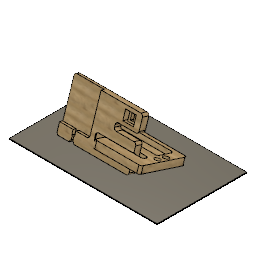
Phone Stand Valet Thingy (Autodesk Fusion 360 design; units mm, degrees)
Autodesk Fusion 360 part; units mm, degrees
note: some values were not read from the file. Set by a fixed rule: which sketch regions a step uses.
sketch "Face Plate Sketch" plane through (0, 0, 0) normal (0, 0, 1) x (1, 0, 0)
  line L0 (6.35, 0) -> (196.85, 0)
  line L1 (196.85, 136.525) -> (6.35, 136.525)
  line L2 (0, 130.175) -> (0, 6.35)
  line L3 (0, 28.575) -> (77.7875, 28.575)
  line L4 (84.1375, 34.925) -> (84.1375, 136.525)
  line L5 (196.85, 92.075) -> (146.05, 92.075)
  line L6 (139.7, 92.075) -> (139.7, 136.525)
  line L7 (139.7, 85.725) -> (139.7, 79.375)
  line L8 (146.05, 73.025) -> (196.85, 73.025)
  line L9 (203.2, 50.165) -> (103.1875, 50.165)
  line L10 (96.8375, 43.815) -> (96.8375, 34.925)
  line L11 (103.1875, 28.575) -> (203.2, 28.575)
  line L12 (203.2, 6.35) -> (203.2, 66.675)
  line L13 (203.2, 98.425) -> (203.2, 130.175)
  arc A0 (146.05, 92.075) -> (139.7, 85.725) centre (146.05, 85.725) ccw
  arc A1 (196.85, 92.075) -> (203.2, 98.425) centre (196.85, 98.425) ccw
  arc A2 (203.2, 130.175) -> (196.85, 136.525) centre (196.85, 130.175) ccw
  arc A3 (139.7, 79.375) -> (146.05, 73.025) centre (146.05, 79.375) ccw
  arc A4 (203.2, 66.675) -> (196.85, 73.025) centre (196.85, 66.675) ccw
  arc A5 (103.1875, 50.165) -> (96.8375, 43.815) centre (103.1875, 43.815) ccw
  arc A6 (96.8375, 34.925) -> (103.1875, 28.575) centre (103.1875, 34.925) ccw
  arc A7 (196.85, 0) -> (203.2, 6.35) centre (196.85, 6.35) ccw
  arc A8 (0, 6.35) -> (6.35, 0) centre (6.35, 6.35) ccw
  arc A9 (6.35, 136.525) -> (0, 130.175) centre (6.35, 130.175) ccw
  arc A10 (77.7875, 28.575) -> (84.1375, 34.925) centre (77.7875, 34.925) ccw
  line L14 (139.7, 114.3) -> (171.45, 114.3) construction
  line L15 (171.45, 92.075) -> (171.45, 127) construction
  line L16 (171.45, 114.3) -> (203.2, 114.3) construction
  line L17 (175.4188, 122.2375) -> (167.4813, 122.2375)
  line L18 (167.4813, 122.2375) -> (167.4813, 106.3625)
  line L19 (167.4813, 106.3625) -> (175.4188, 106.3625)
  line L20 (175.4188, 106.3625) -> (175.4188, 122.2375)
  line L21 (175.4188, 122.2375) -> (167.4813, 106.3625) construction
  line L22 (167.4813, 122.2375) -> (175.4188, 106.3625) construction
  line L23 (181.3719, 103.1875) -> (161.5281, 103.1875)
  line L24 (161.5281, 103.1875) -> (161.5281, 125.4125)
  line L25 (161.5281, 125.4125) -> (181.3719, 125.4125)
  line L26 (181.3719, 125.4125) -> (181.3719, 103.1875)
  line L27 (181.3719, 103.1875) -> (161.5281, 125.4125) construction
  line L28 (161.5281, 103.1875) -> (181.3719, 125.4125) construction
  line L29 (186.5313, 101.2031) -> (156.3688, 101.2031)
  line L30 (156.3688, 101.2031) -> (156.3688, 127.3969)
  line L31 (156.3688, 127.3969) -> (186.5313, 127.3969)
  line L32 (186.5313, 127.3969) -> (186.5313, 101.2031)
  line L33 (186.5313, 101.2031) -> (156.3688, 127.3969) construction
  line L34 (156.3688, 101.2031) -> (186.5313, 127.3969) construction
  line L35 (161.5281, 125.4125) -> (161.5281, 127.3969)
  line L36 (181.3719, 125.4125) -> (181.3719, 127.3969)
  line L37 (181.3719, 103.1875) -> (181.3719, 101.2031)
  line L38 (161.5281, 103.1875) -> (161.5281, 101.2031)
  line L39 (42.0687, 31.8116) -> (42.0687, 28.575) construction
  line L40 (38.1, 28.575) -> (46.0375, 28.575)
  line L41 (46.0375, 28.575) -> (46.0375, 16.6687)
  line L42 (46.0375, 16.6687) -> (38.1, 16.6687)
  line L43 (38.1, 16.6687) -> (38.1, 28.575)
  line L44 (44.2531, 16.6687) -> (39.8843, 16.6687)
  line L45 (39.8843, 16.6687) -> (39.8843, 5.5562)
  line L46 (39.8843, 5.5562) -> (44.2531, 5.5562)
  line L47 (44.2531, 5.5562) -> (44.2531, 16.6687)
  line L48 (40.4812, 5.5562) -> (43.6562, 5.5562)
  line L49 (43.6562, 5.5562) -> (43.6563, 0)
  line L50 (43.6563, 0) -> (40.4813, 0)
  line L51 (40.4813, 0) -> (40.4812, 5.5562)
  line L52 (40.4813, 0) -> (43.6563, 0)
  circle A11 centre (42.0688, 0) radius 6.35
  point P0 (203.2, 0)
  point P1 (84.1375, 28.575)
  point P2 (139.7, 73.025)
  point P3 (96.8375, 50.165)
  point P4 (96.8375, 28.575)
  point P5 (171.45, 114.3)
  point P6 (171.45, 114.3)
  point P7 (171.45, 114.3)
  point P8 (171.45, 114.3)
  point P9 (42.0687, 28.575)
  point P10 (42.0687, 16.6687)
  point P11 (42.0687, 16.6687)
  point P12 (42.0687, 5.5562)
  point P13 (42.0687, 5.5562)
  point P14 (42.0688, 0)
  dimension "d3" = 84.1375
  dimension "d5" = 44.45
  dimension "d6" = 19.05
  dimension "d8" = 12.7
  dimension "d9" = 21.59
  dimension "d12" = 28.575
  dimension "d13" = 25.4
  dimension "d28" = 6.35
  dimension "d29" = 6.35
  dimension "d30" = 6.35
  dimension "d31" = 6.35
  dimension "d32" = 6.35
  dimension "d33" = 6.35
  dimension "d76" = 106.3625
  dimension "d77" = 203.2
  dimension "d163" = 6.35
  dimension "d185" = 63.5
  dimension "d193" = 7.9375
  dimension "d194" = 15.875
  dimension "d195" = 19.8438
  dimension "d196" = 22.225
  dimension "d197" = 26.1938
  dimension "d198" = 30.1625
  dimension "d202" = 7.9375
  dimension "d203" = 11.9062
  dimension "d204" = 11.1125
  dimension "d205" = 4.3688
  dimension "d206" = 3.175
  dimension "d220" = 12.7
  dimension "d224" = 136.525
  measures "d3" distance of L3.start P1
  measures "d5" distance of L6.start L6.end
  measures "d6" distance of L6.start P2
  measures "d8" distance of L4 L10
  measures "d9" distance of P3 P4
  measures "d12" distance of L0 L11
  measures "d28" radius of A0
  measures "d29" radius of A1
  measures "d30" radius of A3
  measures "d31" radius of A5
  measures "d32" radius of A7
  measures "d33" radius of A10
  measures "d76" distance of L10 L12
  measures "d77" distance of L2 L12
  measures "d163" radius of A9
  measures "d185" distance of L6 L13
  measures "d193" distance of L17.start L17.end
  measures "d194" distance of L17.end L18.end
  measures "d195" distance of L24.end L25.end
  measures "d196" distance of L23.end L24.end
  measures "d197" distance of L29.end L30.end
  measures "d198" distance of L30.end L31.end
  measures "d202" distance of L40.start L40.end
  measures "d203" distance of L40.start L42.end
  measures "d204" distance of L44.start L46.end
  measures "d205" distance of L44.start L44.end
  measures "d206" distance of L48.start L48.end
  measures "d220" diameter of A11
  measures "d224" distance of L0 L1
extrude "Extrude1" add sketch "Face Plate Sketch" along normal blind 19.05 contours L0 L2 L3 A8 L42 L43 L45 A11 | L0 L1 L3 L4 L5 L7 L8 L9 L10 L11 L12 L13 A0 A1 A2 A3 A4 A5 A6 A7 A10 L41 L42 L47 A11 makes body 1 at (108.7286, 91.0847, 0) makes body 2 at (12.7, 17.1979, 0) in component "Face Plate"
extrude "Extrude6" add sketch "Face Plate Sketch" along normal blind 9.525 contours L42 L44 L45 L47 A11 | L3 L40 L41 L42 L43 L44 bodies 1 2 in component "Face Plate"
extrude "Extrude2" add sketch "Face Plate Sketch" along normal blind 15.875 contours L9 L10 L11 L12 A5 A6 bodies 1 in component "Face Plate"
extrude "Extrude4" add sketch "Face Plate Sketch" along normal blind 9.525 contours L1 L2 L3 L4 A9 A10 L40 bodies 1 in component "Face Plate"
extrude "Extrude5" add sketch "Face Plate Sketch" along normal blind 10.16 contours L23 L29 L37 L38 | L23 L24 L25 L26 | L25 L31 L35 L36 bodies 1 in component "Face Plate"
sketch "iPhone" plane through (0, 0, 0) normal (0, 0, 1) x (1, 0, 0)
  line L0 (0, 0) -> (77.724, 0)
  line L1 (77.724, 0) -> (77.724, 157.988)
  line L2 (77.724, 157.988) -> (0, 157.988)
  line L3 (0, 157.988) -> (0, 0)
  dimension "d49" = 157.988
  dimension "d50" = 77.724
  measures "d49" distance of L0.start L2.end
  measures "d50" distance of L1.end L2.end
extrude "Extrude1'" add sketch "iPhone" along normal blind 7.112 separate body makes body 3 in component "iPhone"
sketch "Base Plate Sketch" plane through (0, 0, 0) normal (0, 1, 0) x (1, 0, 0)
  line L0 (0, 0) -> (119.0625, 0)
  line L1 (125.4125, 6.35) -> (125.4125, 130.175)
  line L2 (119.0625, 136.525) -> (-71.4375, 136.525)
  line L3 (-6.35, 31.75) -> (93.6625, 31.75)
  line L4 (100.0125, 38.1) -> (100.0125, 42.8625)
  line L5 (93.6625, 49.2125) -> (-71.4375, 49.2125)
  arc A0 (93.6625, 31.75) -> (100.0125, 38.1) centre (93.6625, 38.1) ccw
  arc A1 (100.0125, 42.8625) -> (93.6625, 49.2125) centre (93.6625, 42.8625) ccw
  line L6 (-77.7875, 130.175) -> (-77.7875, 55.5625)
  line L7 (-6.35, 31.75) -> (-6.35, 6.35)
  circle A2 centre (112.7125, 87.3125) radius 7.9375
  arc A3 (-6.35, 6.35) -> (0, 0) centre (0, 6.35) ccw
  arc A4 (119.0625, 0) -> (125.4125, 6.35) centre (119.0625, 6.35) ccw
  arc A5 (125.4125, 130.175) -> (119.0625, 136.525) centre (119.0625, 130.175) ccw
  arc A6 (-71.4375, 136.525) -> (-77.7875, 130.175) centre (-71.4375, 130.175) ccw
  arc A7 (-77.7875, 55.5625) -> (-71.4375, 49.2125) centre (-71.4375, 55.5625) ccw
  line L8 (-58.7375, 123.825) -> (93.6625, 123.825)
  line L9 (100.0125, 117.475) -> (100.0125, 80.9625)
  line L10 (93.6625, 74.6125) -> (-58.7375, 74.6125)
  line L11 (-65.0875, 80.9625) -> (-65.0875, 117.475)
  arc A8 (-58.7375, 123.825) -> (-65.0875, 117.475) centre (-58.7375, 117.475) ccw
  arc A9 (-65.0875, 80.9625) -> (-58.7375, 74.6125) centre (-58.7375, 80.9625) ccw
  arc A10 (93.6625, 74.6125) -> (100.0125, 80.9625) centre (93.6625, 80.9625) ccw
  arc A11 (100.0125, 117.475) -> (93.6625, 123.825) centre (93.6625, 117.475) ccw
  line L12 (112.7125, 61.9125) -> (112.7125, 87.3125) construction
  line L13 (9.525, 65.8813) -> (25.4, 65.8813)
  line L14 (25.4, 65.8813) -> (25.4, 57.9438)
  line L15 (25.4, 57.9438) -> (9.525, 57.9438)
  line L16 (9.525, 57.9438) -> (9.525, 65.8813)
  line L17 (17.4625, 65.8813) -> (17.4625, 74.6125) construction
  line L18 (17.4625, 57.9438) -> (17.4625, 49.2125) construction
  arc A12 (112.4188, 69.8446) -> (113.0062, 53.9804) centre (112.7125, 61.9125) ccw
  arc A13 (113.0062, 53.9804) -> (112.4188, 69.8446) centre (112.7125, 61.9125) ccw
  line L19 (85.4474, 49.2125) -> (85.4474, 74.6125) construction
  line L20 (85.4474, 61.9125) -> (125.4125, 61.9125) construction
  point P0 (125.4125, 0)
  point P1 (125.4125, 136.525)
  point P2 (-77.7875, 136.525)
  point P3 (100.0125, 31.75)
  point P4 (17.4625, 74.6125)
  point P5 (17.4625, 65.8813)
  dimension "d80" = 17.4625
  dimension "d82" = 31.75
  dimension "d83" = 6.35
  dimension "d84" = 6.35
  dimension "d114" = 136.525
  dimension "d115" = 203.2
  dimension "d116" = 25.4
  dimension "d118" = 106.3625
  dimension "d143" = 15.875
  dimension "d144" = 12.7
  dimension "d146" = 6.35
  dimension "d147" = 6.35
  dimension "d148" = 6.35
  dimension "d149" = 6.35
  dimension "d150" = 6.35
  dimension "d151" = 12.7
  dimension "d152" = 25.4
  dimension "d153" = 12.7
  dimension "d154" = 25.4
  dimension "d156" = 6.35
  dimension "d157" = 6.35
  dimension "d158" = 6.35
  dimension "d159" = 6.35
  dimension "d201" = 15.875
  dimension "d221" = 15.875
  dimension "d222" = 7.9375
  dimension "d223" = 25.4
  measures "d80" distance of L3 L5
  measures "d82" distance of L0 L3
  measures "d83" radius of A0
  measures "d84" radius of A1
  measures "d114" distance of P0 P1
  measures "d115" distance of P1 P2
  measures "d116" distance of L1 L4
  measures "d118" distance of L4.end L7
  measures "d143" diameter of A2
  measures "d144" distance of L1 A2.centre
  measures "d146" radius of A3
  measures "d147" radius of A4
  measures "d148" radius of A5
  measures "d149" radius of A6
  measures "d150" radius of A7
  measures "d151" distance of L6 L11
  measures "d152" distance of L1 L9
  measures "d153" distance of L2 L8
  measures "d154" distance of L5 L10
  measures "d156" radius of A8
  measures "d157" radius of A9
  measures "d158" radius of A10
  measures "d159" radius of A11
  measures "d201" diameter of A12
  measures "d221" distance of L13.start L13.end
  measures "d222" distance of L13.start L15.end
  measures "d223" distance of L12.start A2.centre
extrude "Extrude1''" add sketch "Base Plate Sketch" along normal blind 19.05 separate body makes body 4 in component "Base Plate"
extrude "Extrude2'" add sketch "Base Plate Sketch" along normal blind 6.35 contours L8 L9 L10 L11 A8 A9 A10 A11 bodies 4 in component "Base Plate"
box "BoxPrimitive1" add length 254 width 419.1 height 2.54 placed x (0, 0, 1) y (1, 0, 0) z (0, 1, 0) at (-63.5, 0, -101.6) separate body makes body 5 in component "Valet"
copy_body "CutPasteBodies1" bodies 5 removing the originals makes body 6 in component "Ground"
sketch "Base Plate Projection" plane through (105.9656, 43.559, 37.6193) normal (0, 0.951326, -0.308187) x (1, 0, 0)
  circle A0 centre (112.7125, 61.9125) radius 7.9375
  line L0 (25.4, 57.9438) -> (9.525, 57.9438)
  line L1 (9.525, 57.9438) -> (9.525, 65.8813)
  line L2 (9.525, 65.8813) -> (25.4, 65.8813)
  line L3 (25.4, 65.8813) -> (25.4, 57.9438)
  arc A1 (93.6625, 74.6125) -> (100.0125, 80.9625) centre (93.6625, 80.9625) ccw
  line L4 (93.6625, 74.6125) -> (-58.7375, 74.6125)
  arc A2 (-65.0875, 80.9625) -> (-58.7375, 74.6125) centre (-58.7375, 80.9625) ccw
  line L5 (-65.0875, 80.9625) -> (-65.0875, 117.475)
  arc A3 (-58.7375, 123.825) -> (-65.0875, 117.475) centre (-58.7375, 117.475) ccw
  line L6 (-58.7375, 123.825) -> (93.6625, 123.825)
  arc A4 (100.0125, 117.475) -> (93.6625, 123.825) centre (93.6625, 117.475) ccw
  line L7 (100.0125, 117.475) -> (100.0125, 80.9625)
  circle A5 centre (112.7125, 87.3125) radius 7.9375
  line L8 (-6.35, 31.75) -> (-6.35, 6.35)
  arc A6 (-6.35, 6.35) -> (0, 0) centre (0, 6.35) ccw
  line L9 (0, 0) -> (119.0625, 0)
  arc A7 (119.0625, 0) -> (125.4125, 6.35) centre (119.0625, 6.35) ccw
  line L10 (125.4125, 6.35) -> (125.4125, 130.175)
  arc A8 (125.4125, 130.175) -> (119.0625, 136.525) centre (119.0625, 130.175) ccw
  line L11 (119.0625, 136.525) -> (-71.4375, 136.525)
  arc A9 (-71.4375, 136.525) -> (-77.7875, 130.175) centre (-71.4375, 130.175) ccw
  line L12 (-77.7875, 130.175) -> (-77.7875, 55.5625)
  arc A10 (-77.7875, 55.5625) -> (-71.4375, 49.2125) centre (-71.4375, 55.5625) ccw
  line L13 (-71.4375, 49.2125) -> (93.6625, 49.2125)
  arc A11 (100.0125, 42.8625) -> (93.6625, 49.2125) centre (93.6625, 42.8625) ccw
  line L14 (100.0125, 42.8625) -> (100.0125, 38.1)
  arc A12 (93.6625, 31.75) -> (100.0125, 38.1) centre (93.6625, 38.1) ccw
  line L15 (93.6625, 31.75) -> (-6.35, 31.75)
sketch "Face Plate Projection" plane through (0, 0, 0) normal (0, 0.308187, 0.951326) x (1, 0, 0)
  line L0 (156.3688, 127.3969) -> (186.5313, 127.3969)
  line L1 (186.5313, 127.3969) -> (186.5313, 101.2031)
  line L2 (186.5313, 101.2031) -> (156.3688, 101.2031)
  line L3 (156.3688, 101.2031) -> (156.3688, 127.3969)
  arc A0 (196.85, 0) -> (203.2, 6.35) centre (196.85, 6.35) ccw
  line L4 (203.2, 6.35) -> (203.2, 28.575)
  line L5 (203.2, 28.575) -> (103.1875, 28.575)
  arc A1 (96.8375, 34.925) -> (103.1875, 28.575) centre (103.1875, 34.925) ccw
  line L6 (96.8375, 34.925) -> (96.8375, 43.815)
  arc A2 (103.1875, 50.165) -> (96.8375, 43.815) centre (103.1875, 43.815) ccw
  line L7 (103.1875, 50.165) -> (203.2, 50.165)
  line L8 (203.2, 50.165) -> (203.2, 66.675)
  arc A3 (203.2, 66.675) -> (196.85, 73.025) centre (196.85, 66.675) ccw
  line L9 (196.85, 73.025) -> (146.05, 73.025)
  arc A4 (139.7, 79.375) -> (146.05, 73.025) centre (146.05, 79.375) ccw
  line L10 (139.7, 79.375) -> (139.7, 85.725)
  arc A5 (146.05, 92.075) -> (139.7, 85.725) centre (146.05, 85.725) ccw
  line L11 (146.05, 92.075) -> (196.85, 92.075)
  arc A6 (196.85, 92.075) -> (203.2, 98.425) centre (196.85, 98.425) ccw
  line L12 (203.2, 98.425) -> (203.2, 130.175)
  arc A7 (203.2, 130.175) -> (196.85, 136.525) centre (196.85, 130.175) ccw
  line L13 (196.85, 136.525) -> (84.1375, 136.525)
  line L14 (84.1375, 136.525) -> (84.1375, 34.925)
  arc A8 (77.7875, 28.575) -> (84.1375, 34.925) centre (77.7875, 34.925) ccw
  line L15 (77.7875, 28.575) -> (46.0375, 28.575)
  line L16 (46.0375, 28.575) -> (46.0375, 16.6687)
  line L17 (46.0375, 16.6687) -> (44.2531, 16.6687)
  line L18 (44.2531, 16.6687) -> (44.2531, 5.9625)
  arc A9 (48.4188, 0) -> (44.2531, 5.9625) centre (42.0688, 0) ccw
  line L19 (48.4188, 0) -> (196.85, 0)
  arc A10 (96.8375, 34.925) -> (103.1875, 28.575) centre (103.1875, 34.925) ccw
  line L20 (103.1875, 28.575) -> (203.2, 28.575)
  line L21 (203.2, 28.575) -> (203.2, 50.165)
  line L22 (203.2, 50.165) -> (103.1875, 50.165)
  arc A11 (103.1875, 50.165) -> (96.8375, 43.815) centre (103.1875, 43.815) ccw
  line L23 (96.8375, 43.815) -> (96.8375, 34.925)
  line L24 (39.8843, 16.6687) -> (39.8843, 5.9625)
  arc A12 (44.2531, 5.9625) -> (39.8843, 5.9625) centre (42.0688, 0) ccw
  line L25 (44.2531, 5.9625) -> (44.2531, 16.6687)
  line L26 (44.2531, 16.6687) -> (46.0375, 16.6687)
  line L27 (46.0375, 16.6687) -> (46.0375, 28.575)
  line L28 (46.0375, 28.575) -> (77.7875, 28.575)
  arc A13 (77.7875, 28.575) -> (84.1375, 34.925) centre (77.7875, 34.925) ccw
  line L29 (84.1375, 34.925) -> (84.1375, 136.525)
  line L30 (84.1375, 136.525) -> (6.35, 136.525)
  arc A14 (6.35, 136.525) -> (0, 130.175) centre (6.35, 130.175) ccw
  line L31 (0, 130.175) -> (0, 28.575)
  line L32 (0, 28.575) -> (38.1, 28.575)
  line L33 (38.1, 28.575) -> (38.1, 16.6687)
  line L34 (38.1, 16.6687) -> (39.8843, 16.6687)
  line L35 (38.1, 16.6687) -> (38.1, 28.575)
  line L36 (38.1, 28.575) -> (0, 28.575)
  line L37 (0, 28.575) -> (0, 6.35)
  arc A15 (0, 6.35) -> (6.35, 0) centre (6.35, 6.35) ccw
  line L38 (6.35, 0) -> (35.7188, 0)
  arc A16 (39.8843, 5.9625) -> (35.7188, 0) centre (42.0688, 0) ccw
  line L39 (39.8843, 5.9625) -> (39.8843, 16.6687)
  line L40 (39.8843, 16.6687) -> (38.1, 16.6687)
  line L41 (175.4188, 122.2375) -> (175.4188, 106.3625)
  line L42 (175.4188, 106.3625) -> (167.4813, 106.3625)
  line L43 (167.4813, 106.3625) -> (167.4813, 122.2375)
  line L44 (167.4813, 122.2375) -> (175.4188, 122.2375)
  line L45 (161.5281, 127.3969) -> (161.5281, 101.2031)
  line L46 (161.5281, 101.2031) -> (181.3719, 101.2031)
  line L47 (181.3719, 101.2031) -> (181.3719, 127.3969)
  line L48 (181.3719, 127.3969) -> (161.5281, 127.3969)
component "Valet" placed x (1, 0, 0) y (0, 0.951326, -0.308187) z (0, 0.308187, 0.951326) at (0, 0, 0)
component "Ground" placed x (1, 0, 0) y (0, 1, 0) z (0, 0, 1) at (0, -2.54, -63.5)
component "Face Plate" placed x (1, 0, 0) y (0, 1, 0) z (0, 0, 1) at (0, 0, 0) in component "Valet"
component "Base Plate" placed x (1, 0, 0) y (0, 1, 0) z (0, 0, 1) at (127.5933, 29.845, 49.2125) in component "Valet"
component "iPhone" placed x (1, 0, 0) y (0, 1, 0) z (0, 0, 1) at (3.2067, 28.575, 10.7315) in component "Valet"
equation "d3 = 3 5/16\""
equation "d6 = 3/4\""
equation "d12 = 1 1/8\""
equation "d13 = 1\""
equation "d25 = 3/4\""
equation "Fillets = 1/4\""
equation "d28 = Fillets"
equation "d29 = Fillets"
equation "d30 = Fillets"
equation "d31 = Fillets"
equation "d32 = Fillets"
equation "d33 = Fillets"
equation "d37 = 3/4\" - 1/8\""
equation "d53 = 0\""
equation "d54 = 0\""
equation "d55 = 0\""
equation "d57 = 0\""
equation "d58 = 0\""
equation "d59 = 0\""
equation "d62 = 29/32\""
equation "d63 = 0\""
equation "d64 = 0\""
equation "d65 = 0\""
equation "d66 = 0\""
equation "d67 = 0\""
equation "d69 = 0\""
equation "d70 = 0\""
equation "d71 = 0\""
equation "GrooveLen = 4 3/16\""
equation "d76 = GrooveLen"
equation "d77 = 8\""
equation "d80 = 3/4\" - 1/16\""
equation "d82 = 1 1/4\""
equation "d83 = Fillets"
equation "d84 = Fillets"
equation "d85 = ( 3 / 4 ) * 1 in"
equation "d87 = 0\""
equation "d88 = 0\""
equation "d89 = 0\""
equation "d91 = 0\""
equation "d92 = 0\""
equation "d93 = 0\""
equation "d96 = 0\""
equation "d97 = 0\""
equation "d98 = -3/4\" + 1/8\""
equation "d99 = 0\""
equation "d100 = 0\""
equation "d101 = 0\""
equation "d103 = 0\""
equation "d104 = 0\""
equation "d105 = 0\""
equation "d107 = -1 19/64\""
equation "d108 = 2 1/2\""
equation "d109 = 10\""
equation "d110 = 16 1/2\""
equation "d112 = 0\""
equation "d113 = 0\""
equation "d114 = 5.5 in - 0.125 in"
equation "d118 = GrooveLen"
equation "d119 = 0\""
equation "d120 = 0\""
equation "d121 = 0\""
equation "d123 = 0\""
equation "d124 = 0\""
equation "d125 = 0\""
equation "d128 = 0\""
equation "d129 = 0\""
equation "d130 = 0\""
equation "d132 = 0\""
equation "d133 = 0\""
equation "d134 = 0\""
equation "d144 = 1/2\""
equation "d146 = Fillets"
equation "d147 = Fillets"
equation "d148 = Fillets"
equation "d149 = Fillets"
equation "d150 = Fillets"
equation "d156 = Fillets"
equation "d157 = Fillets"
equation "d158 = Fillets"
equation "d159 = Fillets"
equation "d160 = ( 1 / 4 ) * 1 in"
equation "d163 = 1/4\""
equation "d193 = 5/16\""
equation "d194 = 5/8\""
equation "d195 = 3/4\" + 1/32\""
equation "d196 = 7/8\""
equation "d197 = 1 1/32\""
equation "d198 = 1 3/16\""
equation "d199 = 3/4\" - 0.35 in"
equation "d202 = 5/16\""
equation "d203 = 15/32\""
equation "d204 = 7/16\""
equation "d206 = 1/8\""
equation "d210 = 3/8\""
equation "d212 = 0\""
equation "d213 = 0\""
equation "d214 = 0\""
equation "d216 = 0\""
equation "d217 = 0\""
equation "d218 = 0\""
equation "d220 = 1/2\""
equation "d221 = ( 5 / 8 ) * 1 in"
equation "d222 = ( 5 / 16 ) * 1 in"
equation "d224 = 5.50 in - 0.125 in"
